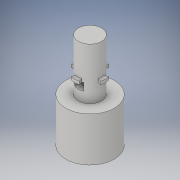
# Autodesk Inventor part: SoportePulgada
Saved by Autodesk Inventor 2019 (Build 230136000, 136)
## iProperties
Created: 2020-03-30
Part Number: SoportePulgada
Material: Generic
Document SubType Name: Modeling
Designer: Sergio
Density: 1 g/cm^3
Appearance: Default
Author: Sergio
Autodesk Inventor part; units mm, degrees
ref_plane "YZ Plane" through (0, 0, 0) normal (1, 0, 0) x (0, 1, 0)
ref_plane "XZ Plane" through (0, 0, 0) normal (0, 1, 0) x (-1, 0, 0)
ref_plane "XY Plane" through (0, 0, 0) normal (0, 0, 1) x (1, 0, 0)
sketch "Sketch1" plane through (0, 0, 0) normal (0, 1, 0) x (-1, 0, 0)
  circle A0 centre (0, 0) radius 7.85
  dimension "d0" = 15.7
  constraints: 1 centre point
  measures "d0" diameter of A0
extrude "Extrusion1" add sketch "Sketch1" along normal blind 35
sketch "Sketch2" plane through (0, 0, 0) normal (0, -1, 0) x (1, 0, 0)
  circle A0 centre (0, 0) radius 16.4
  dimension "d3" = 32.8
  constraints: 1 centre point, 1 coincident
  measures "d3" diameter of A0
extrude "Extrusion2" add sketch "Sketch2" along normal blind 30
sketch "Sketch3" plane through (0, 0, 0) normal (1, 0, 0) x (0, 1, 0)
  line L0 (-30, 16.4) -> (-30, -16.4) projected
  line L1 (7, 4) -> (-30, 4)
  line L2 (-30, 4) -> (-30, -4)
  line L3 (-30, -4) -> (7, -4)
  line L4 (0, 7.85) -> (35, 7.85) projected
  line L5 (0, -7.85) -> (35, -7.85) projected
  line L6 (12, 7.85) -> (7, 7.85)
  line L7 (7, -7.85) -> (12, -7.85)
  line L8 (12, -7.85) -> (12, 7.85)
  line L9 (7, 7.85) -> (7, 4)
  line L10 (7, -4) -> (7, -7.85)
  point P0 (0, 0)
  dimension "d7" = 4
  dimension "d8" = 4
  dimension "d12" = 5
  dimension "d13" = 37
  constraints: 16 end point, 4 parallel, 3 perpendicular, 3 point on line, 2 horizontal
  measures "d7" distance from line of L3 point (0, 0)
  measures "d8" distance from line of point (0, 0) L1
  measures "d12" distance between parallel lines of L10 L8
  measures "d13" distance between parallel lines of L0 L10
extrude "Extrusion3" cut sketch "Sketch3" along normal mid plane 6
sketch "Sketch4" plane through (0, 0, 0) normal (1, 0, 0) x (0, 1, 0)
  line L0 (12, -7.85) -> (12, -7.2541) projected
  line L1 (12, -7.85) -> (14, -7.85)
  line L2 (14, -7.85) -> (14, -10.35)
  line L3 (14, -10.35) -> (12, -10.35)
  line L4 (12, -10.35) -> (12, -7.85)
  line L5 (-2.8, 0) -> (16.8, 0) projected
  point P0 (0, 0)
  dimension "d14" = 2
  dimension "d15" = 2.5
  constraints: 8 end point, 2 parallel, 1 horizontal, 1 perpendicular
  measures "d14" distance of L2.end L3.end
  measures "d15" distance of L1.end L2.end
revolve "Revolution1" add sketch "Sketch4" angle 30 mid plane about axis through (0, -10, 0) along (0, 1, 0)
pattern_circular "Circular Pattern1" count 4 over 360 about axis through (0, -10, 0) along (0, 1, 0) of "Revolution1"
body "Solid1"
